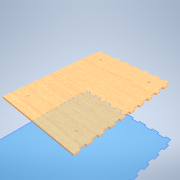
# Autodesk Inventor part: TableBottom
Saved by Autodesk Inventor 2021 (Build 250183000, 183)
## iProperties
Created: 2021-03-11
Part Number: TableBottom
Material: Wood (Cherry)
Document SubType Name: Modeling
Designer: ZiweZhang
Density: 0.63 g/cm^3
Appearance: Cherry - Natural Low Gloss
Author: ZiweZhang
Autodesk Inventor part; units mm, degrees
ref_plane "YZ Plane" through (0, 0, 0) normal (1, 0, 0) x (0, 1, 0)
ref_plane "XZ Plane" through (0, 0, 0) normal (0, 1, 0) x (-1, 0, 0)
ref_plane "XY Plane" through (0, 0, 0) normal (0, 0, 1) x (1, 0, 0)
sketch "Sketch2" plane through (0, 0, 0) normal (0, 1, 0) x (-1, 0, 0)
  line L0 (0, 0) -> (150, 0)
  line L1 (150, 0) -> (150, -200)
  line L2 (150, -200) -> (0, -200)
  line L3 (0, -200) -> (0, 0)
  point P0 (75, -100)
  dimension "d4" = 150
  dimension "d5" = 200
  constraints: 8 end point, 2 parallel, 1 horizontal, 1 perpendicular
  measures "d4" distance of L1.end L2.end
  measures "d5" distance of L0.end L1.end
extrude "Extrusion2" add sketch "Sketch2" along normal blind 3
sketch "Sketch3" plane through (0, 0, 0) normal (0, -1, 0) x (1, 0, 0)
  line L0 (-150, -200) -> (-150, 0) projected
  line L1 (-150, 0) -> (-150, -10)
  line L2 (-150, -10) -> (-147, -10)
  line L3 (-147, -10) -> (-147, -20)
  line L4 (-147, -20) -> (-150, -20)
  line L5 (-147, -30) -> (-147, -40)
  line L6 (-147, -40) -> (-150, -40)
  line L7 (-150, -30) -> (-147, -30)
  line L8 (-150, -20) -> (-150, -30)
  line L9 (-147, -50) -> (-147, -60)
  line L10 (-147, -60) -> (-150, -60)
  line L11 (-150, -50) -> (-147, -50)
  line L12 (-150, -40) -> (-150, -50)
  line L13 (-147, -70) -> (-147, -80)
  line L14 (-147, -80) -> (-150, -80)
  line L15 (-150, -70) -> (-147, -70)
  line L16 (-150, -60) -> (-150, -70)
  line L17 (-147, -90) -> (-147, -100)
  line L18 (-147, -100) -> (-150, -100)
  line L19 (-150, -90) -> (-147, -90)
  line L20 (-150, -80) -> (-150, -90)
  line L21 (-147, -110) -> (-147, -120)
  line L22 (-147, -120) -> (-150, -120)
  line L23 (-150, -110) -> (-147, -110)
  line L24 (-150, -100) -> (-150, -110)
  line L25 (-147, -130) -> (-147, -140)
  line L26 (-147, -140) -> (-150, -140)
  line L27 (-150, -130) -> (-147, -130)
  line L28 (-150, -120) -> (-150, -130)
  line L29 (-147, -150) -> (-147, -160)
  line L30 (-147, -160) -> (-150, -160)
  line L31 (-150, -150) -> (-147, -150)
  line L32 (-150, -140) -> (-150, -150)
  line L33 (-147, -170) -> (-147, -180)
  line L34 (-147, -180) -> (-150, -180)
  line L35 (-150, -170) -> (-147, -170)
  line L36 (-150, -160) -> (-150, -170)
  line L37 (-150, -180) -> (-150, -190)
  line L38 (-150, -190) -> (-147, -190)
  line L39 (0, 0) -> (0, -10)
  line L40 (0, 0) -> (0, -200) projected
  line L41 (-3, -10) -> (-3, -20)
  line L42 (-3, -20) -> (0, -20)
  line L43 (0, -20) -> (0, -30)
  line L44 (0, -30) -> (-3, -30)
  line L45 (-3, -30) -> (-3, -40)
  line L46 (-3, -40) -> (0, -40)
  line L47 (0, -40) -> (0, -50)
  line L48 (0, -50) -> (-3, -50)
  line L49 (-3, -50) -> (-3, -60)
  line L50 (-3, -60) -> (0, -60)
  line L51 (0, -60) -> (0, -70)
  line L52 (0, -70) -> (-3, -70)
  line L53 (-3, -70) -> (-3, -80)
  line L54 (-3, -80) -> (0, -80)
  line L55 (0, -80) -> (0, -90)
  line L56 (0, -90) -> (-3, -90)
  line L57 (-3, -90) -> (-3, -100)
  line L58 (-3, -100) -> (0, -100)
  line L59 (0, -100) -> (0, -110)
  line L60 (0, -110) -> (-3, -110)
  line L61 (-3, -110) -> (-3, -120)
  line L62 (-3, -120) -> (0, -120)
  line L63 (0, -120) -> (0, -130)
  line L64 (0, -130) -> (-3, -130)
  line L65 (-3, -130) -> (-3, -140)
  line L66 (-3, -140) -> (0, -140)
  line L67 (0, -140) -> (0, -150)
  line L68 (0, -150) -> (-3, -150)
  line L69 (-3, -150) -> (-3, -160)
  line L70 (-3, -160) -> (0, -160)
  line L71 (0, -160) -> (0, -170)
  line L72 (0, -170) -> (-3, -170)
  line L73 (-3, -170) -> (-3, -180)
  line L74 (-3, -180) -> (0, -180)
  line L75 (0, -180) -> (0, -190)
  line L76 (0, -190) -> (-3, -190)
  line L77 (-3, -190) -> (-3, -200)
  line L78 (0, -200) -> (-150, -200) projected
  line L79 (-147, -190) -> (-147, -200)
  line L80 (0, -10) -> (-3, -10)
  line L81 (-147, -200) -> (-140, -200)
  line L82 (-140, -197) -> (-130, -197)
  line L83 (-130, -197) -> (-130, -200)
  line L84 (-120, -200) -> (-120, -197)
  line L85 (-120, -197) -> (-110, -197)
  line L86 (-110, -197) -> (-110, -200)
  line L87 (-100, -200) -> (-100, -197)
  line L88 (-100, -197) -> (-90, -197)
  line L89 (-90, -197) -> (-90, -200)
  line L90 (-80, -200) -> (-80, -197)
  line L91 (-80, -197) -> (-70, -197)
  line L92 (-70, -197) -> (-70, -200)
  line L93 (-60, -200) -> (-60, -197)
  line L94 (-60, -197) -> (-50, -197)
  line L95 (-50, -197) -> (-50, -200)
  line L96 (-40, -200) -> (-40, -197)
  line L97 (-40, -197) -> (-30, -197)
  line L98 (-30, -197) -> (-30, -200)
  line L99 (-20, -200) -> (-20, -197)
  line L100 (-20, -197) -> (-10, -197)
  line L101 (-10, -197) -> (-10, -200)
  line L102 (-140, -197) -> (-140, -200)
  line L103 (-150, 0) -> (0, 0)
  point P0 (-10, 0)
  point P1 (-20, 0)
  dimension "d23" = 20
  constraints: 202 end point, 48 point on line, 40 vertical alignment, 24 perpendicular, 18 parallel, 16 collinear, 12 vertical, 3 horizontal, 23 other
  measures "d23" distance of L2.end L5.start
extrude "Extrusion3" cut sketch "Sketch3" against normal blind 3 contours L0 L34 L33 L35 L30 L29 L31 L26 L25 L27 L22 L21 L23 L18 L17 L19 L14 L13 L15 L10 L9 L11 L6 L5 L7 L4 L3 L2 L103 L39 L80 L41 L42 L40 L44 L45 L46 L48 L49 L50 L52 L53 L54 L56 L57 L58 L60 L61 L62 L64 L65 L66 L68 L69 L70 L72 L73 L74 L76 L77 L78 L101 L100 L99 L98 L97 L96 L95 L94 L93 L92 L91 L90 L89 L88 L87 L86 L85 L84 L83 L82 L102 L79 L38 keep common part
sketch "Sketch5" plane through (0, 3, 0) normal (0, 1, 0) x (1, 0, 0)
  line L0 (-150, 190) -> (-150, 0) projected
  circle A0 centre (-24.8562, 25.4431) radius 2.5
  circle A1 centre (-124.8562, 25.4431) radius 2.5
  circle A2 centre (-24.8562, 175.4431) radius 2.5
  circle A3 centre (-124.8562, 175.4431) radius 2.5
  point P0 (0, 0)
  point P1 (-150, 10)
  point P2 (0, 0)
  point P3 (-75, 100)
  dimension "d38" = 5
  dimension "d39" = 100
  dimension "d40" = 150
  constraints: 4 centre point
  measures "d38" diameter of A0
  measures "d39" distance of A0.centre A1.centre
  measures "d40" distance of A0.centre A2.centre
extrude "Extrusion4" cut sketch "Sketch5" against normal blind 2
body "Solid2"
